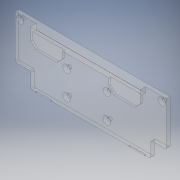
# Autodesk Inventor part: OdriveMountingBracket
Saved by Autodesk Inventor 2019.3 (Build 233278000, 278)
## iProperties
Created: 2019-02-15
Part Number: OdriveMountingBracket
Material: PET Plastic
Document SubType Name: Modeling
Designer: mark
Density: 1.541 g/cm^3
Appearance: Polycarbonate - Clear
Author: mark
Autodesk Inventor part; units mm, degrees
ref_plane "YZ Plane" through (0, 0, 0) normal (1, 0, 0) x (0, 1, 0)
ref_plane "XZ Plane" through (0, 0, 0) normal (0, 1, 0) x (-1, 0, 0)
ref_plane "XY Plane" through (0, 0, 0) normal (0, 0, 1) x (1, 0, 0)
sketch "Sketch1" plane through (0, 0, 0) normal (0, 0, 1) x (1, 0, 0)
  circle A0 centre (138, -2.5) radius 1.7
  circle A1 centre (2.5, -2.5) radius 1.7
  circle A2 centre (47, -20.9) radius 1.7
  circle A3 centre (85.5, -20.9) radius 1.7
  circle A4 centre (85.5, -20.9) radius 1.7
  circle A5 centre (47, -20.9) radius 1.7
  circle A6 centre (2.5, -2.5) radius 1.7
  circle A7 centre (138, -2.5) radius 1.7
  line L0 (0, 0) -> (0, -2.7254)
  circle A8 centre (85.5, -44.5) radius 1.7
  circle A9 centre (85.5, -44.5) radius 1.7
  circle A10 centre (47, -44.5) radius 1.7
  line L1 (-2, 2) -> (142.5, 2)
  line L2 (127.5, -55) -> (13, -55)
  line L3 (-2, 2) -> (-2, -40)
  line L4 (-2, -40) -> (13, -40)
  line L5 (13, -40) -> (13, -55)
  line L6 (142.5, 2) -> (142.5, -40)
  line L7 (142.5, -40) -> (127.5, -40)
  line L8 (127.5, -40) -> (127.5, -55)
  dimension "d37" = 47
  dimension "d46" = 2.5
  dimension "d49" = 3.4
  dimension "d50" = 3.4
  dimension "d51" = 3.4
  dimension "d52" = 3.4
  dimension "d53" = 3.4
  dimension "d54" = 3.4
  dimension "d57" = 47
  dimension "d62" = 15
  dimension "d63" = 15
  dimension "d64" = 15
  dimension "d65" = 15
  constraints: 18 end point, 11 centre point, 6 coincident, 5 vertical, 2 horizontal
  measures "d37" distance from line of L0 A2.centre
  measures "d46" distance from line of L0 A1.centre
  measures "d49" diameter of A1
  measures "d50" diameter of A2
  measures "d51" diameter of A3
  measures "d52" diameter of A8
  measures "d53" diameter of A10
  measures "d54" diameter of A0
  measures "d57" distance from line of L0 A10.centre
  measures "d62" distance between parallel lines of L3 L5
  measures "d63" distance between parallel lines of L6 L8
  measures "d64" distance between parallel lines of L2 L7
  measures "d65" distance between parallel lines of L2 L4
extrude "Extrusion1" add sketch "Sketch1" along normal blind 3.5
sketch "Sketch5" plane through (0, 0, 3.5) normal (0, 0, 1) x (1, 0, 0)
  line L0 (-2, -40) -> (-2, 2) projected
  line L1 (142.5, 2) -> (142.5, -40) projected
  line L2 (122.5, 2) -> (18, 2)
  line L3 (18, 2) -> (18, 0)
  line L4 (18, 0) -> (122.5, 0)
  line L5 (122.5, 0) -> (122.5, 2)
  line L6 (142.5, 2) -> (-2, 2) projected
  point P0 (142.5, 0)
  dimension "d101" = 2
  dimension "d102" = 20
  dimension "d103" = 20
  constraints: 8 end point, 1 collinear, 1 point on line
  measures "d101" distance between parallel lines of L2 L4
  measures "d102" distance between parallel lines of L0 L3
  measures "d103" distance between parallel lines of L5 L1
extrude "Extrusion5" add sketch "Sketch5" along normal blind 5.1
sketch "Sketch6" plane through (0, 0, 3.5) normal (0, 0, 1) x (1, 0, 0)
  line L0 (18, -54) -> (33, -54)
  line L1 (33, -54) -> (33, -55)
  line L2 (33, -55) -> (18, -55)
  line L3 (18, -55) -> (18, -54)
  line L4 (107.5, -54) -> (122.5, -54)
  line L5 (122.5, -54) -> (122.5, -55)
  line L6 (122.5, -55) -> (107.5, -55)
  line L7 (107.5, -55) -> (107.5, -54)
  line L8 (-2, 0) -> (142.5, 0) projected
  line L9 (13, -40) -> (13, -55) projected
  line L10 (127.5, -55) -> (127.5, -40) projected
  line L11 (13, -55) -> (127.5, -55) projected
  point P0 (0, 0)
  dimension "d69" = 1
  dimension "d70" = 15
  dimension "d71" = 5
  dimension "d73" = 15
  dimension "d74" = 5
  constraints: 16 end point, 3 collinear
  measures "d69" distance between parallel lines of L2 L0
  measures "d70" distance between parallel lines of L3 L1
  measures "d71" distance between parallel lines of L9 L3
  measures "d73" distance between parallel lines of L7 L5
  measures "d74" distance between parallel lines of L10 L5
extrude "Extrusion6" add sketch "Sketch6" along normal blind 1
fillet "Fillet3" radius 0.5 4 edges at (25.5, -55, 4.5) (25.5, -54, 4.5) (115, -54, 4.5) (115, -55, 4.5)
sketch "Sketch7" plane through (3, 0, 3.5) normal (0, -1, 0) x (1, 0, 0)
  line L0 (15, 3.2) -> (45, 3.2)
  line L1 (45, 3.2) -> (45, 5.1)
  line L2 (45, 5.1) -> (15, 5.1)
  line L3 (15, 5.1) -> (15, 3.2)
  line L4 (89.5, 3.2) -> (119.5, 3.2)
  line L5 (119.5, 3.2) -> (119.5, 5.1)
  line L6 (119.5, 5.1) -> (89.5, 5.1)
  line L7 (89.5, 5.1) -> (89.5, 3.2)
  line L8 (10, 0) -> (124.5, 0) projected
  line L9 (-5, -3.5) -> (-5, 0) projected
  line L10 (139.5, -3.5) -> (139.5, 0) projected
  point P0 (-3, -3.5)
  dimension "d78" = 3.2
  dimension "d80" = 30
  dimension "d82" = 30
  dimension "d106" = 20
  dimension "d107" = 20
  constraints: 16 end point, 1 collinear
  measures "d78" distance between parallel lines of L8 L0
  measures "d80" distance between parallel lines of L1 L3
  measures "d82" distance between parallel lines of L7 L5
  measures "d106" distance between parallel lines of L3 L9
  measures "d107" distance between parallel lines of L5 L10
extrude "Extrusion7" add sketch "Sketch7" along normal blind 15
chamfer "Chamfer2" distance 5 angle 45 4 edges at (48, -15, 7.65) (18, -15, 7.65) (92.5, -15, 7.65) (122.5, -15, 7.65)
chamfer "Chamfer3" distance 1 angle 45 6 edges at (13, -55, 1.75) (13, -40, 1.75) (-2, -40, 1.75) (127.5, -55, 1.75) (142.5, -40, 1.75) (127.5, -40, 1.75)
chamfer "Chamfer4" distance 2 angle 45 6 edges at (0.8, -2.5, 3.5) (45.3, -20.9, 3.5) (45.3, -44.5, 3.5) (83.8, -44.5, 3.5) (83.8, -20.9, 3.5) (136.3, -2.5, 3.5)
sketch "Sketch8" plane through (53, 0, 8.6) normal (0, -1, 0) x (1, 0, 0)
  line L0 (-35, -1.9) -> (69.5, -1.9)
  line L1 (69.5, -1.9) -> (69.5, -5.1)
  line L2 (69.5, -5.1) -> (-35, -5.1)
  line L3 (-35, -5.1) -> (-35, -1.9)
  line L4 (-20, -5.1) -> (54.5, -5.1) projected
  line L5 (-30, -1.9) -> (-10, -1.9) projected
  line L6 (-55, -5.1) -> (-55, -8.6) projected
  line L7 (89.5, -8.6) -> (89.5, -5.1) projected
  point P0 (-53, -8.6)
  dimension "d108" = 20
  dimension "d109" = 20
  constraints: 8 end point, 2 collinear
  measures "d108" distance between parallel lines of L6 L3
  measures "d109" distance between parallel lines of L7 L1
extrude "Extrusion8" add sketch "Sketch8" along normal blind 3.25
sketch "Sketch10" plane through (48, 0, 6.7) normal (0, 0, 1) x (1, 0, 0)
  line L0 (44.5, 0) -> (44.5, -3.25) projected
  line L1 (0, 0) -> (44.5, 0) projected
  line L2 (0, 0) -> (0, -3.25) projected
  line L3 (44.5, -3.25) -> (0, -3.25) projected
  line L4 (44.5, 0) -> (0, 0)
  line L5 (0, 0) -> (0, -3.25)
  line L6 (0, -3.25) -> (44.5, -3.25)
  line L7 (44.5, -3.25) -> (44.5, 0)
  point P0 (-48, 0)
  constraints: 8 end point
extrude "Extrusion9" add sketch "Sketch10" along normal up to surface (1.9 mm away)
body "Solid1"
